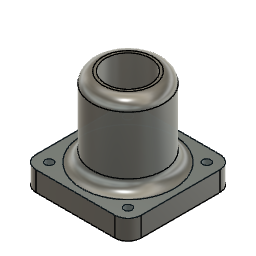
TDP3SensorOccluder (Autodesk Fusion 360 design; units mm, degrees)
Autodesk Fusion 360 part; units mm, degrees
sketch "Sketch1" plane through (0, 0, 0) normal (0, 1, 0) x (1, 0, 0)
  line L0 (15, 20) -> (-15, 20)
  line L1 (-20, 15) -> (-20, -15)
  line L2 (-15, -20) -> (15, -20)
  line L3 (20, -15) -> (20, 15)
  line L4 (20, 20) -> (-20, -20) construction
  line L5 (-20, 20) -> (20, -20) construction
  arc A0 (20, 15) -> (15, 20) centre (15, 15) ccw
  arc A1 (-20, -15) -> (-15, -20) centre (-15, -15) ccw
  arc A2 (15, -20) -> (20, -15) centre (15, -15) ccw
  arc A3 (-15, 20) -> (-20, 15) centre (-15, 15) ccw
  circle A4 centre (-15, 15) radius 1.55
  circle A5 centre (15, 15) radius 1.55
  circle A6 centre (15, -15) radius 1.55
  circle A7 centre (-15, -15) radius 1.55
  circle A8 centre (0, 0) radius 8.5
  dimension "d1" = 40
  dimension "d2" = 5
  dimension "d4" = 3.1
  dimension "d5" = 17
  constraint horizontal L0
  constraint perpendicular L0 L1
  constraint parallel L0 L2
  constraint parallel L1 L3
  constraint coincident L4 A8.centre
  constraint coincident L5 A8.centre
  constraint coincident A8.centre origin
  constraint coincident L4.start L0
  constraint coincident L4.start L3
  constraint tangent L0 A0
  constraint tangent L3 A0
  constraint coincident L4.end L2
  constraint coincident L4.end L1
  constraint tangent L2 A1
  constraint tangent L1 A1
  constraint equal A0 A1
  constraint coincident L5.end L3
  constraint coincident L5.end L2
  constraint tangent L3 A2
  constraint tangent L2 A2
  constraint equal A0 A2
  constraint coincident L5.start L0
  constraint coincident L5.start L1
  constraint tangent L0 A3
  constraint tangent L1 A3
  constraint equal A0 A3
  constraint equal L0 L1
  constraint concentric A3 A4
  constraint concentric A0 A5
  constraint concentric A2 A6
  constraint concentric A1 A7
  constraint equal A4 A5
  constraint equal A5 A6
  constraint equal A6 A7
  measures "d1" distance of L4.start L5.start
  measures "d2" radius of A0
  measures "d4" diameter of A4
  measures "d5" diameter of A8
extrude "Extrude1" add sketch "Sketch1" along normal blind 7.5
sketch "Sketch2" plane through (0, 7.5, 0) normal (0, 1, 0) x (-1, 0, 0)
  circle A0 centre (15, -15) radius 1.55
  circle A1 centre (-15, -15) radius 1.55
  circle A2 centre (-15, 15) radius 1.55
  circle A3 centre (15, 15) radius 1.55
  circle A4 centre (0, 0) radius 8.5
  arc A5 (15, -20) -> (20, -15) centre (15, -15) ccw
  line L0 (20, -15) -> (20, 15)
  arc A6 (20, 15) -> (15, 20) centre (15, 15) ccw
  line L1 (15, 20) -> (-15, 20)
  arc A7 (-15, 20) -> (-20, 15) centre (-15, 15) ccw
  line L2 (-20, 15) -> (-20, -15)
  arc A8 (-20, -15) -> (-15, -20) centre (-15, -15) ccw
  line L3 (-15, -20) -> (15, -20)
  circle A9 centre (0, 0) radius 8.5
  circle A10 centre (0, 0) radius 13.5
  dimension "d8" = 5
  constraint coincident A4.centre A9.centre
  constraint concentric A9 A10
  constraint tangent A4 A9
  measures "d8" distance of A9 A10
extrude "Extrude2" add sketch "Sketch2" along normal blind 30 contours A10
fillet "Fillet1" radius 4 1 faces at (-13.4329, 27.5, -1.3442)
sketch "Sketch3" plane through (0, 7.5, 0) normal (0, 1, 0) x (-1, 0, 0)
  arc A0 (15, -20) -> (20, -15) centre (15, -15) ccw
  line L0 (20, -15) -> (20, 15)
  arc A1 (20, 15) -> (15, 20) centre (15, 15) ccw
  line L1 (15, 20) -> (-15, 20)
  arc A2 (-15, 20) -> (-20, 15) centre (-15, 15) ccw
  line L2 (-20, 15) -> (-20, -15)
  arc A3 (-20, -15) -> (-15, -20) centre (-15, -15) ccw
  line L3 (-15, -20) -> (15, -20)
  circle A4 centre (15, 15) radius 1.55
  circle A5 centre (-15, -15) radius 1.55
  circle A6 centre (15, -15) radius 1.55
  circle A7 centre (-15, 15) radius 1.55
  circle A8 centre (0, 0) radius 17.5
